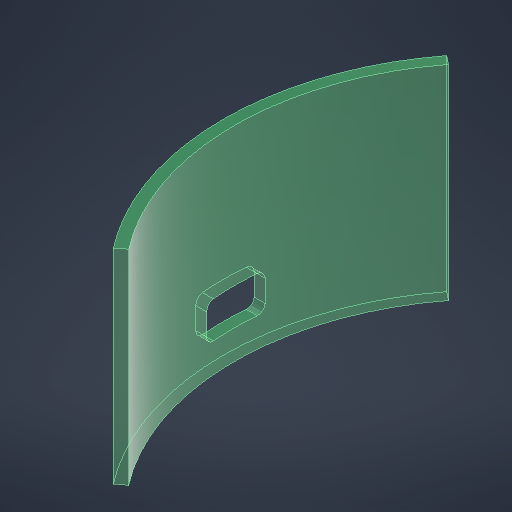
# Autodesk Inventor part: PARED TRASERA
Saved by Autodesk Inventor 2026.2 (Build 302298000, 298)
## iProperties
Created: 2026-02-05
Part Number: PARED TRASERA
Material: Generic
Document SubType Name: Modeling
Designer: 06aar
Density: 1 g/cm^3
Appearance: Clear - Green 1
Author: 06aar
Autodesk Inventor part; units mm, degrees
ref_plane "YZ Plane" through (0, 0, 0) normal (1, 0, 0) x (0, 1, 0)
ref_plane "XZ Plane" through (0, 0, 0) normal (0, 1, 0) x (-1, 0, 0)
ref_plane "XY Plane" through (0, 0, 0) normal (0, 0, 1) x (1, 0, 0)
sketch "Sketch1" plane through (0, 0, 0) normal (0, 1, 0) x (-1, 0, 0)
  circle A0 centre (0, 0) radius 75
  circle A1 centre (0, 0) radius 72
  line L0 (0, 0) -> (59.5015, -45.6571)
  line L1 (0, 0) -> (59.5015, 45.6571)
  line L2 (0, 0) -> (75, 0)
  arc A2 (58.3115, -44.744) -> (58.3115, 44.744) centre (0, 0) ccw
  point P0 (57.1214, 43.8308)
  point P1 (57.1214, -43.8308)
  dimension "d0" = 150
  dimension "d1" = 3
  dimension "d2" = 37.5
  dimension "d3" = 37.5
  dimension "d13" = 1.5
  constraints: 6 end point, 5 point on circle, 3 centre point, 3 coincident, 2 point on line, 1 horizontal
  measures "d0" diameter of A0
  measures "d1" radial gap between concentric circles of A0 A1
  measures "d2" angle of L2 L1
  measures "d3" angle of L2 L0
  measures "d13" radial gap between concentric circles of A1 A2
extrude "Extrusion1" add sketch "Sketch1" along normal blind 56 contours L2 A2 L1 A0 | A0 L0 A2 L2 | A2 L0 A1 L2 | L2 A1 L1 A2
sketch "Sketch2" plane through (0, 0, 0) normal (1, 0, 0) x (0, 1, 0)
  line L0 (8, 0) -> (18, 0)
  line L1 (18, 0) -> (18, 6)
  line L2 (16, 8) -> (10, 8)
  line L3 (8, 6) -> (8, 0)
  line L4 (8, 0) -> (18, 0)
  line L5 (18, 0) -> (18, -6)
  line L6 (16, -8) -> (10, -8)
  line L7 (8, -6) -> (8, 0)
  line L8 (0, -45.6571) -> (0, 45.6571) projected
  line L9 (0, 0) -> (8, 0)
  arc A0 (16, -8) -> (18, -6) centre (16, -6) ccw
  arc A1 (18, 6) -> (16, 8) centre (16, 6) ccw
  arc A2 (10, 8) -> (8, 6) centre (10, 6) ccw
  arc A3 (8, -6) -> (10, -8) centre (10, -6) ccw
  point P0 (18, 8)
  point P1 (8, 8)
  point P2 (18, -8)
  point P3 (8, -8)
  dimension "d6" = 8
  dimension "d7" = 8
  dimension "d8" = 10
  dimension "d12" = 2
  constraints: 18 end point, 9 point on line, 8 point on circle, 8 tangent, 4 centre point, 4 parallel, 3 equal radius, 3 horizontal, 2 perpendicular, 1 collinear
  measures "d6" distance of point (8, -8) L0.start
  measures "d7" distance between parallel lines of L3 L8
  measures "d8" distance of point (18, 8) point (8, 8)
  measures "d12" radius of A0
extrude "Extrusion2" cut sketch "Sketch2" against normal blind 100
body "Solid1"
